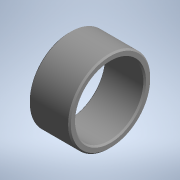
# Autodesk Inventor part: WSSS12-10-6
Saved by Autodesk Inventor 2020 (Build 240168000, 168)
## iProperties
Part Number: WSSS12-10-6
Material: 一般
Catalog Web Link: www.cadenas.de
Description: WSSB, WSSM, WSSS,WSSA,WSSAB-Metal Washers - Standard Class - T Dimension Selectable -
Vendor: MISUMI
Document SubType Name: Modeling
Designer: partserver
Manufacturer: MISUMI
Mass: 0.204581 g
Surface Area: 4.67611 cm^2
Volume: 0.204581 cm^3
Density: 1 g/cm^3
Appearance: PSOLRGB-175-175-175
Category: PARTsolutions
Company: MISUMI
PSOL_IDENT_0: {$CADENAS_DATA\23d-libs\misumi\metric\26_washers_collars\wssb.prj},197 {VTYP=3D},{NB=WSSS12-10-6},{L
PSOL_IDENT_1: INA=WSSS12-10-6},{NN=WSSB, WSSM, WSSS,WSSA,WSSAB},{DATE=07.06.2021 12:12:34},{GEOMDATE=20.01.2021 07
PSOL_IDENT_2: :37:58},{VERSION=},{LINEID=250},{WBVAR=MAT,ST,V,T},{WBNUMERIC=V,T}  {NB=WSSS12-10-6},{LINA=WSSS12-10
PSOL_IDENT_3: -6},{KT=DUMMY},{PN=WSSS12-10-6},{TYPE=WSSS},{MAT=304},{MATALG= '1045', '1045 Carbon Steel', '304', '
PSOL_IDENT_4: 304 Stainless Steel', '2000',' 2000 aluminum alloy' },{ST=-},{STALG= '-','-' },{DALG=4,5,6,8,10,12,1
PSOL_IDENT_5: 3,14,15,16,20,25,30,35,40,50,60},{D=12},{V=10},{VALG=3,4,5,6,8,10},{VALG1=3,4,5,6,8,10},{VALG2=0},{T=
PSOL_IDENT_6: 6.0},{TALG=1,1.5,2,2.5,3,4,5,6,8},{TALG1=1,1.5,2,2.5,3,4,5,6,8},{TALG2=1,2,3,5},{C=0.2}
NB: WSSS12-10-6
NN: WSSB, WSSM, WSSS,WSSA,WSSAB
NT: Metal Washers - Standard Class - T Dimension Selectable -
NBSYN: $PN.
LINA: WSSS12-10-6
CATALOG: Misumi
PN: WSSS12-10-6
MAT: 304 Stainless Steel
ST: -
D: 12
V: 10
T: 6
SUPPLIER: MISUMI
ARTICLENO: WSSS12-10-6
BOMINFO: WSSS12-10-6
CREATOR: CADENAS GmbH
Title: WSSS12-10-6
Author: Cadenas PARTsolutions
Comments: Metal Washers - Standard Class - T Dimension Selectable -
Autodesk Inventor part; units mm, degrees
sketch "Sketch_1" plane through (0, 0, 0) normal (0, 0, 1) x (1, 0, 0)
  line L0 (-3, 0) -> (3, 0)
  line L1 (0, -5.2) -> (0, -5.8)
  line L2 (0, -5.8) -> (0.2, -6)
  line L3 (0.2, -6) -> (5.8, -6)
  line L4 (5.8, -6) -> (6, -5.8)
  line L5 (6, -5.8) -> (6, -5.2)
  line L6 (6, -5.2) -> (5.8, -5)
  line L7 (5.8, -5) -> (0.2, -5)
  line L8 (0.2, -5) -> (0, -5.2)
  constraints: 18 end point
revolve "Revolution1" add sketch "Sketch_1" angle 360 about axis through (-3, 0, 0) along (-1, 0, 0)
ref_plane "a_XY" through (0, 0, 0) normal (1, 0, 0) x (0, 0, -1)
ref_plane "a_YZ" through (0, 0, 0) normal (0, 0, -1) x (0, 1, 0)
ref_plane "a_ZX" through (0, 0, 0) normal (0, 1, 0) x (1, 0, 0)
body "Solid1"
